Autodesk Inventor part; units mm, degrees
note: some values were not read from the file. Chosen so that the rebuilt part matches the saved one: sketch regions of "LensplateMount".
(part 2 of 2)
sketch "ShorterHoneycomb" plane through (93.9578, 0, 52.0444) normal (1, 0, 0) x (0, 0, -1)
  line L0 (0, 131) -> (119, 131)
  line L1 (119, 131) -> (119, 0)
  line L2 (119, 0) -> (0, 0)
  line L3 (0, 0) -> (0, 131)
  line L4 (7, 131) -> (112, 131)
  line L5 (112, 131) -> (112, 0)
  line L6 (112, 0) -> (7, 0)
  line L7 (7, 0) -> (7, 131)
  line L8 (21.8083, 115) -> (14.3028, 115)
  line L9 (14.3028, 115) -> (10.55, 121.5)
  line L10 (10.55, 121.5) -> (14.3028, 128)
  line L11 (14.3028, 128) -> (21.8083, 128)
  line L12 (21.8083, 128) -> (25.5611, 121.5)
  line L13 (25.5611, 121.5) -> (21.8083, 115)
  line L14 (33.644, 107.5) -> (26.1385, 107.5)
  line L15 (26.1385, 107.5) -> (22.3857, 114)
  line L16 (22.3857, 114) -> (26.1385, 120.5)
  line L17 (26.1385, 120.5) -> (33.644, 120.5)
  line L18 (33.644, 120.5) -> (37.3968, 114)
  line L19 (37.3968, 114) -> (33.644, 107.5)
  line L20 (0, 131) -> (119, 131) projected
  line L21 (25.5611, 121.5) -> (26.1385, 120.5) construction
  line L22 (21.8083, 115) -> (22.3857, 114) construction
  line L23 (21.8083, 100) -> (14.3028, 100)
  line L24 (14.3028, 100) -> (10.55, 106.5)
  line L25 (10.55, 106.5) -> (14.3028, 113)
  line L26 (14.3028, 113) -> (21.8083, 113)
  line L27 (21.8083, 113) -> (25.5611, 106.5)
  line L28 (25.5611, 106.5) -> (21.8083, 100)
  line L29 (33.644, 92.5) -> (26.1385, 92.5)
  line L30 (26.1385, 92.5) -> (22.3857, 99)
  line L31 (22.3857, 99) -> (26.1385, 105.5)
  line L32 (26.1385, 105.5) -> (33.644, 105.5)
  line L33 (33.644, 105.5) -> (37.3968, 99)
  line L34 (37.3968, 99) -> (33.644, 92.5)
  line L35 (25.5611, 106.5) -> (26.1385, 105.5) construction
  line L36 (21.8083, 100) -> (22.3857, 99) construction
  line L37 (21.8083, 85) -> (14.3028, 85)
  line L38 (14.3028, 85) -> (10.55, 91.5)
  line L39 (10.55, 91.5) -> (14.3028, 98)
  line L40 (14.3028, 98) -> (21.8083, 98)
  line L41 (21.8083, 98) -> (25.5611, 91.5)
  line L42 (25.5611, 91.5) -> (21.8083, 85)
  line L43 (33.644, 77.5) -> (26.1385, 77.5)
  line L44 (26.1385, 77.5) -> (22.3857, 84)
  line L45 (22.3857, 84) -> (26.1385, 90.5)
  line L46 (26.1385, 90.5) -> (33.644, 90.5)
  line L47 (33.644, 90.5) -> (37.3968, 84)
  line L48 (37.3968, 84) -> (33.644, 77.5)
  line L49 (25.5611, 91.5) -> (26.1385, 90.5) construction
  line L50 (21.8083, 85) -> (22.3857, 84) construction
  line L51 (21.8083, 70) -> (14.3028, 70)
  line L52 (14.3028, 70) -> (10.55, 76.5)
  line L53 (10.55, 76.5) -> (14.3028, 83)
  line L54 (14.3028, 83) -> (21.8083, 83)
  line L55 (21.8083, 83) -> (25.5611, 76.5)
  line L56 (25.5611, 76.5) -> (21.8083, 70)
  line L57 (33.644, 62.5) -> (26.1385, 62.5)
  line L58 (26.1385, 62.5) -> (22.3857, 69)
  line L59 (22.3857, 69) -> (26.1385, 75.5)
  line L60 (26.1385, 75.5) -> (33.644, 75.5)
  line L61 (33.644, 75.5) -> (37.3968, 69)
  line L62 (37.3968, 69) -> (33.644, 62.5)
  line L63 (25.5611, 76.5) -> (26.1385, 75.5) construction
  line L64 (21.8083, 70) -> (22.3857, 69) construction
  line L65 (21.8083, 55) -> (14.3028, 55)
  line L66 (14.3028, 55) -> (10.55, 61.5)
  line L67 (10.55, 61.5) -> (14.3028, 68)
  line L68 (14.3028, 68) -> (21.8083, 68)
  line L69 (21.8083, 68) -> (25.5611, 61.5)
  line L70 (25.5611, 61.5) -> (21.8083, 55)
  line L71 (33.644, 47.5) -> (26.1385, 47.5)
  line L72 (26.1385, 47.5) -> (22.3857, 54)
  line L73 (22.3857, 54) -> (26.1385, 60.5)
  line L74 (26.1385, 60.5) -> (33.644, 60.5)
  line L75 (33.644, 60.5) -> (37.3968, 54)
  line L76 (37.3968, 54) -> (33.644, 47.5)
  line L77 (25.5611, 61.5) -> (26.1385, 60.5) construction
  line L78 (21.8083, 55) -> (22.3857, 54) construction
  line L79 (21.8083, 40) -> (14.3028, 40)
  line L80 (14.3028, 40) -> (10.55, 46.5)
  line L81 (10.55, 46.5) -> (14.3028, 53)
  line L82 (14.3028, 53) -> (21.8083, 53)
  line L83 (21.8083, 53) -> (25.5611, 46.5)
  line L84 (25.5611, 46.5) -> (21.8083, 40)
  line L85 (33.644, 32.5) -> (26.1385, 32.5)
  line L86 (26.1385, 32.5) -> (22.3857, 39)
  line L87 (22.3857, 39) -> (26.1385, 45.5)
  line L88 (26.1385, 45.5) -> (33.644, 45.5)
  line L89 (33.644, 45.5) -> (37.3968, 39)
  line L90 (37.3968, 39) -> (33.644, 32.5)
  line L91 (25.5611, 46.5) -> (26.1385, 45.5) construction
  line L92 (21.8083, 40) -> (22.3857, 39) construction
  line L93 (21.8083, 25) -> (14.3028, 25)
  line L94 (14.3028, 25) -> (10.55, 31.5)
  line L95 (10.55, 31.5) -> (14.3028, 38)
  line L96 (14.3028, 38) -> (21.8083, 38)
  line L97 (21.8083, 38) -> (25.5611, 31.5)
  line L98 (25.5611, 31.5) -> (21.8083, 25)
  line L99 (33.644, 17.5) -> (26.1385, 17.5)
  line L100 (26.1385, 17.5) -> (22.3857, 24)
  line L101 (22.3857, 24) -> (26.1385, 30.5)
  line L102 (26.1385, 30.5) -> (33.644, 30.5)
  line L103 (33.644, 30.5) -> (37.3968, 24)
  line L104 (37.3968, 24) -> (33.644, 17.5)
  line L105 (25.5611, 31.5) -> (26.1385, 30.5) construction
  line L106 (21.8083, 25) -> (22.3857, 24) construction
  line L107 (21.8083, 10) -> (14.3028, 10)
  line L108 (14.3028, 10) -> (10.55, 16.5)
  line L109 (10.55, 16.5) -> (14.3028, 23)
  line L110 (14.3028, 23) -> (21.8083, 23)
  line L111 (21.8083, 23) -> (25.5611, 16.5)
  line L112 (25.5611, 16.5) -> (21.8083, 10)
  line L113 (33.644, 2.5) -> (26.1385, 2.5)
  line L114 (26.1385, 2.5) -> (22.3857, 9)
  line L115 (22.3857, 9) -> (26.1385, 15.5)
  line L116 (26.1385, 15.5) -> (33.644, 15.5)
  line L117 (33.644, 15.5) -> (37.3968, 9)
  line L118 (37.3968, 9) -> (33.644, 2.5)
  line L119 (25.5611, 16.5) -> (26.1385, 15.5) construction
  line L120 (21.8083, 10) -> (22.3857, 9) construction
  line L121 (45.4833, 115) -> (37.9778, 115)
  line L122 (37.9778, 115) -> (34.225, 121.5)
  line L123 (34.225, 121.5) -> (37.9778, 128)
  line L124 (37.9778, 128) -> (45.4833, 128)
  line L125 (45.4833, 128) -> (49.2361, 121.5)
  line L126 (49.2361, 121.5) -> (45.4833, 115)
  line L127 (57.319, 107.5) -> (49.8135, 107.5)
  line L128 (49.8135, 107.5) -> (46.0607, 114)
  line L129 (46.0607, 114) -> (49.8135, 120.5)
  line L130 (49.8135, 120.5) -> (57.319, 120.5)
  line L131 (57.319, 120.5) -> (61.0718, 114)
  line L132 (61.0718, 114) -> (57.319, 107.5)
  line L133 (49.2361, 121.5) -> (49.8135, 120.5) construction
  line L134 (45.4833, 115) -> (46.0607, 114) construction
  line L135 (45.4833, 100) -> (37.9778, 100)
  line L136 (37.9778, 100) -> (34.225, 106.5)
  line L137 (34.225, 106.5) -> (37.9778, 113)
  line L138 (37.9778, 113) -> (45.4833, 113)
  line L139 (45.4833, 113) -> (49.2361, 106.5)
  line L140 (49.2361, 106.5) -> (45.4833, 100)
  line L141 (57.319, 92.5) -> (49.8135, 92.5)
  line L142 (49.8135, 92.5) -> (46.0607, 99)
  line L143 (46.0607, 99) -> (49.8135, 105.5)
  line L144 (49.8135, 105.5) -> (57.319, 105.5)
  line L145 (57.319, 105.5) -> (61.0718, 99)
  line L146 (61.0718, 99) -> (57.319, 92.5)
  line L147 (49.2361, 106.5) -> (49.8135, 105.5) construction
  line L148 (45.4833, 100) -> (46.0607, 99) construction
  line L149 (45.4833, 85) -> (37.9778, 85)
  line L150 (37.9778, 85) -> (34.225, 91.5)
  line L151 (34.225, 91.5) -> (37.9778, 98)
  line L152 (37.9778, 98) -> (45.4833, 98)
  line L153 (45.4833, 98) -> (49.2361, 91.5)
  line L154 (49.2361, 91.5) -> (45.4833, 85)
  line L155 (57.319, 77.5) -> (49.8135, 77.5)
  line L156 (49.8135, 77.5) -> (46.0607, 84)
  line L157 (46.0607, 84) -> (49.8135, 90.5)
  line L158 (49.8135, 90.5) -> (57.319, 90.5)
  line L159 (57.319, 90.5) -> (61.0718, 84)
  line L160 (61.0718, 84) -> (57.319, 77.5)
  line L161 (49.2361, 91.5) -> (49.8135, 90.5) construction
  line L162 (45.4833, 85) -> (46.0607, 84) construction
  line L163 (45.4833, 70) -> (37.9778, 70)
  line L164 (37.9778, 70) -> (34.225, 76.5)
  line L165 (34.225, 76.5) -> (37.9778, 83)
  line L166 (37.9778, 83) -> (45.4833, 83)
  line L167 (45.4833, 83) -> (49.2361, 76.5)
  line L168 (49.2361, 76.5) -> (45.4833, 70)
  line L169 (57.319, 62.5) -> (49.8135, 62.5)
  line L170 (49.8135, 62.5) -> (46.0607, 69)
  line L171 (46.0607, 69) -> (49.8135, 75.5)
  line L172 (49.8135, 75.5) -> (57.319, 75.5)
  line L173 (57.319, 75.5) -> (61.0718, 69)
  line L174 (61.0718, 69) -> (57.319, 62.5)
  line L175 (49.2361, 76.5) -> (49.8135, 75.5) construction
  line L176 (45.4833, 70) -> (46.0607, 69) construction
  line L177 (45.4833, 55) -> (37.9778, 55)
  line L178 (37.9778, 55) -> (34.225, 61.5)
  line L179 (34.225, 61.5) -> (37.9778, 68)
  line L180 (37.9778, 68) -> (45.4833, 68)
  line L181 (45.4833, 68) -> (49.2361, 61.5)
  line L182 (49.2361, 61.5) -> (45.4833, 55)
  line L183 (57.319, 47.5) -> (49.8135, 47.5)
  line L184 (49.8135, 47.5) -> (46.0607, 54)
  line L185 (46.0607, 54) -> (49.8135, 60.5)
  line L186 (49.8135, 60.5) -> (57.319, 60.5)
  line L187 (57.319, 60.5) -> (61.0718, 54)
  line L188 (61.0718, 54) -> (57.319, 47.5)
  line L189 (49.2361, 61.5) -> (49.8135, 60.5) construction
  line L190 (45.4833, 55) -> (46.0607, 54) construction
  line L191 (45.4833, 40) -> (37.9778, 40)
  line L192 (37.9778, 40) -> (34.225, 46.5)
  line L193 (34.225, 46.5) -> (37.9778, 53)
  line L194 (37.9778, 53) -> (45.4833, 53)
  line L195 (45.4833, 53) -> (49.2361, 46.5)
  line L196 (49.2361, 46.5) -> (45.4833, 40)
  line L197 (57.319, 32.5) -> (49.8135, 32.5)
  line L198 (49.8135, 32.5) -> (46.0607, 39)
  line L199 (46.0607, 39) -> (49.8135, 45.5)
  line L200 (49.8135, 45.5) -> (57.319, 45.5)
  line L201 (57.319, 45.5) -> (61.0718, 39)
  line L202 (61.0718, 39) -> (57.319, 32.5)
  line L203 (49.2361, 46.5) -> (49.8135, 45.5) construction
  line L204 (45.4833, 40) -> (46.0607, 39) construction
  line L205 (45.4833, 25) -> (37.9778, 25)
  line L206 (37.9778, 25) -> (34.225, 31.5)
  line L207 (34.225, 31.5) -> (37.9778, 38)
  line L208 (37.9778, 38) -> (45.4833, 38)
  line L209 (45.4833, 38) -> (49.2361, 31.5)
  line L210 (49.2361, 31.5) -> (45.4833, 25)
  line L211 (57.319, 17.5) -> (49.8135, 17.5)
  line L212 (49.8135, 17.5) -> (46.0607, 24)
  line L213 (46.0607, 24) -> (49.8135, 30.5)
  line L214 (49.8135, 30.5) -> (57.319, 30.5)
  line L215 (57.319, 30.5) -> (61.0718, 24)
  line L216 (61.0718, 24) -> (57.319, 17.5)
  line L217 (49.2361, 31.5) -> (49.8135, 30.5) construction
  line L218 (45.4833, 25) -> (46.0607, 24) construction
  line L219 (45.4833, 10) -> (37.9778, 10)
  line L220 (37.9778, 10) -> (34.225, 16.5)
  line L221 (34.225, 16.5) -> (37.9778, 23)
  line L222 (37.9778, 23) -> (45.4833, 23)
  line L223 (45.4833, 23) -> (49.2361, 16.5)
  line L224 (49.2361, 16.5) -> (45.4833, 10)
  line L225 (57.319, 2.5) -> (49.8135, 2.5)
  line L226 (49.8135, 2.5) -> (46.0607, 9)
  line L227 (46.0607, 9) -> (49.8135, 15.5)
  line L228 (49.8135, 15.5) -> (57.319, 15.5)
  line L229 (57.319, 15.5) -> (61.0718, 9)
  line L230 (61.0718, 9) -> (57.319, 2.5)
  line L231 (49.2361, 16.5) -> (49.8135, 15.5) construction
  line L232 (45.4833, 10) -> (46.0607, 9) construction
  line L233 (69.1583, 115) -> (61.6528, 115)
  line L234 (61.6528, 115) -> (57.9, 121.5)
  line L235 (57.9, 121.5) -> (61.6528, 128)
  line L236 (61.6528, 128) -> (69.1583, 128)
  line L237 (69.1583, 128) -> (72.9111, 121.5)
  line L238 (72.9111, 121.5) -> (69.1583, 115)
  line L239 (80.994, 107.5) -> (73.4885, 107.5)
  line L240 (73.4885, 107.5) -> (69.7357, 114)
  line L241 (69.7357, 114) -> (73.4885, 120.5)
  line L242 (73.4885, 120.5) -> (80.994, 120.5)
  line L243 (80.994, 120.5) -> (84.7468, 114)
  line L244 (84.7468, 114) -> (80.994, 107.5)
  line L245 (72.9111, 121.5) -> (73.4885, 120.5) construction
  line L246 (69.1583, 115) -> (69.7357, 114) construction
  line L247 (69.1583, 100) -> (61.6528, 100)
  line L248 (61.6528, 100) -> (57.9, 106.5)
  line L249 (57.9, 106.5) -> (61.6528, 113)
  line L250 (61.6528, 113) -> (69.1583, 113)
  line L251 (69.1583, 113) -> (72.9111, 106.5)
  line L252 (72.9111, 106.5) -> (69.1583, 100)
  line L253 (80.994, 92.5) -> (73.4885, 92.5)
  line L254 (73.4885, 92.5) -> (69.7357, 99)
  line L255 (69.7357, 99) -> (73.4885, 105.5)
  line L256 (73.4885, 105.5) -> (80.994, 105.5)
  line L257 (80.994, 105.5) -> (84.7468, 99)
  line L258 (84.7468, 99) -> (80.994, 92.5)
  line L259 (72.9111, 106.5) -> (73.4885, 105.5) construction
  line L260 (69.1583, 100) -> (69.7357, 99) construction
  line L261 (69.1583, 85) -> (61.6528, 85)
  line L262 (61.6528, 85) -> (57.9, 91.5)
  line L263 (57.9, 91.5) -> (61.6528, 98)
  line L264 (61.6528, 98) -> (69.1583, 98)
  line L265 (69.1583, 98) -> (72.9111, 91.5)
  line L266 (72.9111, 91.5) -> (69.1583, 85)
  line L267 (80.994, 77.5) -> (73.4885, 77.5)
  line L268 (73.4885, 77.5) -> (69.7357, 84)
  line L269 (69.7357, 84) -> (73.4885, 90.5)
  line L270 (73.4885, 90.5) -> (80.994, 90.5)
  line L271 (80.994, 90.5) -> (84.7468, 84)
  line L272 (84.7468, 84) -> (80.994, 77.5)
  line L273 (72.9111, 91.5) -> (73.4885, 90.5) construction
  line L274 (69.1583, 85) -> (69.7357, 84) construction
  line L275 (69.1583, 70) -> (61.6528, 70)
  line L276 (61.6528, 70) -> (57.9, 76.5)
  line L277 (57.9, 76.5) -> (61.6528, 83)
  line L278 (61.6528, 83) -> (69.1583, 83)
  line L279 (69.1583, 83) -> (72.9111, 76.5)
  line L280 (72.9111, 76.5) -> (69.1583, 70)
  line L281 (80.994, 62.5) -> (73.4885, 62.5)
  line L282 (73.4885, 62.5) -> (69.7357, 69)
  line L283 (69.7357, 69) -> (73.4885, 75.5)
  line L284 (73.4885, 75.5) -> (80.994, 75.5)
  line L285 (80.994, 75.5) -> (84.7468, 69)
  line L286 (84.7468, 69) -> (80.994, 62.5)
  line L287 (72.9111, 76.5) -> (73.4885, 75.5) construction
  line L288 (69.1583, 70) -> (69.7357, 69) construction
  line L289 (69.1583, 55) -> (61.6528, 55)
  line L290 (61.6528, 55) -> (57.9, 61.5)
  line L291 (57.9, 61.5) -> (61.6528, 68)
  line L292 (61.6528, 68) -> (69.1583, 68)
  line L293 (69.1583, 68) -> (72.9111, 61.5)
  line L294 (72.9111, 61.5) -> (69.1583, 55)
  line L295 (80.994, 47.5) -> (73.4885, 47.5)
  line L296 (73.4885, 47.5) -> (69.7357, 54)
  line L297 (69.7357, 54) -> (73.4885, 60.5)
  line L298 (73.4885, 60.5) -> (80.994, 60.5)
  line L299 (80.994, 60.5) -> (84.7468, 54)
  line L300 (84.7468, 54) -> (80.994, 47.5)
  line L301 (72.9111, 61.5) -> (73.4885, 60.5) construction
  line L302 (69.1583, 55) -> (69.7357, 54) construction
  line L303 (69.1583, 40) -> (61.6528, 40)
  line L304 (61.6528, 40) -> (57.9, 46.5)
  line L305 (57.9, 46.5) -> (61.6528, 53)
  line L306 (61.6528, 53) -> (69.1583, 53)
  line L307 (69.1583, 53) -> (72.9111, 46.5)
  line L308 (72.9111, 46.5) -> (69.1583, 40)
  line L309 (80.994, 32.5) -> (73.4885, 32.5)
  line L310 (73.4885, 32.5) -> (69.7357, 39)
  line L311 (69.7357, 39) -> (73.4885, 45.5)
  line L312 (73.4885, 45.5) -> (80.994, 45.5)
  line L313 (80.994, 45.5) -> (84.7468, 39)
  line L314 (84.7468, 39) -> (80.994, 32.5)
  line L315 (72.9111, 46.5) -> (73.4885, 45.5) construction
  line L316 (69.1583, 40) -> (69.7357, 39) construction
  line L317 (69.1583, 25) -> (61.6528, 25)
  line L318 (61.6528, 25) -> (57.9, 31.5)
  line L319 (57.9, 31.5) -> (61.6528, 38)
  line L320 (61.6528, 38) -> (69.1583, 38)
  line L321 (69.1583, 38) -> (72.9111, 31.5)
  line L322 (72.9111, 31.5) -> (69.1583, 25)
  line L323 (80.994, 17.5) -> (73.4885, 17.5)
  line L324 (73.4885, 17.5) -> (69.7357, 24)
  line L325 (69.7357, 24) -> (73.4885, 30.5)
  line L326 (73.4885, 30.5) -> (80.994, 30.5)
  line L327 (80.994, 30.5) -> (84.7468, 24)
  line L328 (84.7468, 24) -> (80.994, 17.5)
  line L329 (72.9111, 31.5) -> (73.4885, 30.5) construction
  line L330 (69.1583, 25) -> (69.7357, 24) construction
  line L331 (69.1583, 10) -> (61.6528, 10)
  line L332 (61.6528, 10) -> (57.9, 16.5)
  line L333 (57.9, 16.5) -> (61.6528, 23)
  line L334 (61.6528, 23) -> (69.1583, 23)
  line L335 (69.1583, 23) -> (72.9111, 16.5)
  line L336 (72.9111, 16.5) -> (69.1583, 10)
  line L337 (80.994, 2.5) -> (73.4885, 2.5)
  line L338 (73.4885, 2.5) -> (69.7357, 9)
  line L339 (69.7357, 9) -> (73.4885, 15.5)
  line L340 (73.4885, 15.5) -> (80.994, 15.5)
  line L341 (80.994, 15.5) -> (84.7468, 9)
  line L342 (84.7468, 9) -> (80.994, 2.5)
  line L343 (72.9111, 16.5) -> (73.4885, 15.5) construction
  line L344 (69.1583, 10) -> (69.7357, 9) construction
  line L345 (92.8333, 115) -> (85.3278, 115)
  line L346 (85.3278, 115) -> (81.575, 121.5)
  line L347 (81.575, 121.5) -> (85.3278, 128)
  line L348 (85.3278, 128) -> (92.8333, 128)
  line L349 (92.8333, 128) -> (96.5861, 121.5)
  line L350 (96.5861, 121.5) -> (92.8333, 115)
  line L351 (104.669, 107.5) -> (97.1635, 107.5)
  line L352 (97.1635, 107.5) -> (93.4107, 114)
  line L353 (93.4107, 114) -> (97.1635, 120.5)
  line L354 (97.1635, 120.5) -> (104.669, 120.5)
  line L355 (104.669, 120.5) -> (108.4218, 114)
  line L356 (108.4218, 114) -> (104.669, 107.5)
  line L357 (96.5861, 121.5) -> (97.1635, 120.5) construction
  line L358 (92.8333, 115) -> (93.4107, 114) construction
  line L359 (92.8333, 100) -> (85.3278, 100)
  line L360 (85.3278, 100) -> (81.575, 106.5)
  line L361 (81.575, 106.5) -> (85.3278, 113)
  line L362 (85.3278, 113) -> (92.8333, 113)
  line L363 (92.8333, 113) -> (96.5861, 106.5)
  line L364 (96.5861, 106.5) -> (92.8333, 100)
  line L365 (104.669, 92.5) -> (97.1635, 92.5)
  line L366 (97.1635, 92.5) -> (93.4107, 99)
  line L367 (93.4107, 99) -> (97.1635, 105.5)
  line L368 (97.1635, 105.5) -> (104.669, 105.5)
  line L369 (104.669, 105.5) -> (108.4218, 99)
  line L370 (108.4218, 99) -> (104.669, 92.5)
  line L371 (96.5861, 106.5) -> (97.1635, 105.5) construction
  line L372 (92.8333, 100) -> (93.4107, 99) construction
  line L373 (92.8333, 85) -> (85.3278, 85)
  line L374 (85.3278, 85) -> (81.575, 91.5)
  line L375 (81.575, 91.5) -> (85.3278, 98)
  line L376 (85.3278, 98) -> (92.8333, 98)
  line L377 (92.8333, 98) -> (96.5861, 91.5)
  line L378 (96.5861, 91.5) -> (92.8333, 85)
  line L379 (104.669, 77.5) -> (97.1635, 77.5)
  line L380 (97.1635, 77.5) -> (93.4107, 84)
  line L381 (93.4107, 84) -> (97.1635, 90.5)
  line L382 (97.1635, 90.5) -> (104.669, 90.5)
  line L383 (104.669, 90.5) -> (108.4218, 84)
  line L384 (108.4218, 84) -> (104.669, 77.5)
  line L385 (96.5861, 91.5) -> (97.1635, 90.5) construction
  line L386 (92.8333, 85) -> (93.4107, 84) construction
  line L387 (92.8333, 70) -> (85.3278, 70)
  line L388 (85.3278, 70) -> (81.575, 76.5)
  line L389 (81.575, 76.5) -> (85.3278, 83)
  line L390 (85.3278, 83) -> (92.8333, 83)
  line L391 (92.8333, 83) -> (96.5861, 76.5)
  line L392 (96.5861, 76.5) -> (92.8333, 70)
  line L393 (104.669, 62.5) -> (97.1635, 62.5)
  line L394 (97.1635, 62.5) -> (93.4107, 69)
  line L395 (93.4107, 69) -> (97.1635, 75.5)
  line L396 (97.1635, 75.5) -> (104.669, 75.5)
  line L397 (104.669, 75.5) -> (108.4218, 69)
  line L398 (108.4218, 69) -> (104.669, 62.5)
  line L399 (96.5861, 76.5) -> (97.1635, 75.5) construction
  line L400 (92.8333, 70) -> (93.4107, 69) construction
  line L401 (92.8333, 55) -> (85.3278, 55)
  line L402 (85.3278, 55) -> (81.575, 61.5)
  line L403 (81.575, 61.5) -> (85.3278, 68)
  line L404 (85.3278, 68) -> (92.8333, 68)
  line L405 (92.8333, 68) -> (96.5861, 61.5)
  line L406 (96.5861, 61.5) -> (92.8333, 55)
  line L407 (104.669, 47.5) -> (97.1635, 47.5)
  line L408 (97.1635, 47.5) -> (93.4107, 54)
  line L409 (93.4107, 54) -> (97.1635, 60.5)
  line L410 (97.1635, 60.5) -> (104.669, 60.5)
  line L411 (104.669, 60.5) -> (108.4218, 54)
  line L412 (108.4218, 54) -> (104.669, 47.5)
  line L413 (96.5861, 61.5) -> (97.1635, 60.5) construction
  line L414 (92.8333, 55) -> (93.4107, 54) construction
  line L415 (92.8333, 40) -> (85.3278, 40)
  line L416 (85.3278, 40) -> (81.575, 46.5)
  line L417 (81.575, 46.5) -> (85.3278, 53)
  line L418 (85.3278, 53) -> (92.8333, 53)
  line L419 (92.8333, 53) -> (96.5861, 46.5)
  line L420 (96.5861, 46.5) -> (92.8333, 40)
  line L421 (104.669, 32.5) -> (97.1635, 32.5)
  line L422 (97.1635, 32.5) -> (93.4107, 39)
  line L423 (93.4107, 39) -> (97.1635, 45.5)
  line L424 (97.1635, 45.5) -> (104.669, 45.5)
  line L425 (104.669, 45.5) -> (108.4218, 39)
  line L426 (108.4218, 39) -> (104.669, 32.5)
  line L427 (96.5861, 46.5) -> (97.1635, 45.5) construction
  line L428 (92.8333, 40) -> (93.4107, 39) construction
  line L429 (92.8333, 25) -> (85.3278, 25)
  line L430 (85.3278, 25) -> (81.575, 31.5)
  line L431 (81.575, 31.5) -> (85.3278, 38)
  line L432 (85.3278, 38) -> (92.8333, 38)
  line L433 (92.8333, 38) -> (96.5861, 31.5)
  line L434 (96.5861, 31.5) -> (92.8333, 25)
  line L435 (104.669, 17.5) -> (97.1635, 17.5)
  line L436 (97.1635, 17.5) -> (93.4107, 24)
  line L437 (93.4107, 24) -> (97.1635, 30.5)
  line L438 (97.1635, 30.5) -> (104.669, 30.5)
  line L439 (104.669, 30.5) -> (108.4218, 24)
  line L440 (108.4218, 24) -> (104.669, 17.5)
  line L441 (96.5861, 31.5) -> (97.1635, 30.5) construction
  line L442 (92.8333, 25) -> (93.4107, 24) construction
  line L443 (92.8333, 10) -> (85.3278, 10)
  line L444 (85.3278, 10) -> (81.575, 16.5)
  line L445 (81.575, 16.5) -> (85.3278, 23)
  line L446 (85.3278, 23) -> (92.8333, 23)
  line L447 (92.8333, 23) -> (96.5861, 16.5)
  line L448 (96.5861, 16.5) -> (92.8333, 10)
  line L449 (104.669, 2.5) -> (97.1635, 2.5)
  line L450 (97.1635, 2.5) -> (93.4107, 9)
  line L451 (93.4107, 9) -> (97.1635, 15.5)
  line L452 (97.1635, 15.5) -> (104.669, 15.5)
  line L453 (104.669, 15.5) -> (108.4218, 9)
  line L454 (108.4218, 9) -> (104.669, 2.5)
  line L455 (96.5861, 16.5) -> (97.1635, 15.5) construction
  line L456 (92.8333, 10) -> (93.4107, 9) construction
  line L457 (116.5083, 115) -> (109.0028, 115)
  line L458 (109.0028, 115) -> (105.25, 121.5)
  line L459 (109.0028, 128) -> (116.5083, 128)
  line L460 (116.5083, 128) -> (120.2611, 121.5)
  line L461 (120.2611, 121.5) -> (116.5083, 115)
  line L462 (105.25, 121.5) -> (109.0028, 128)
  line L463 (116.5083, 100) -> (109.0028, 100)
  line L464 (109.0028, 100) -> (105.25, 106.5)
  line L465 (109.0028, 113) -> (116.5083, 113)
  line L466 (116.5083, 113) -> (120.2611, 106.5)
  line L467 (120.2611, 106.5) -> (116.5083, 100)
  line L468 (105.25, 106.5) -> (109.0028, 113)
  line L469 (116.5083, 85) -> (109.0028, 85)
  line L470 (109.0028, 85) -> (105.25, 91.5)
  line L471 (109.0028, 98) -> (116.5083, 98)
  line L472 (116.5083, 98) -> (120.2611, 91.5)
  line L473 (120.2611, 91.5) -> (116.5083, 85)
  line L474 (105.25, 91.5) -> (109.0028, 98)
  line L475 (116.5083, 70) -> (109.0028, 70)
  line L476 (109.0028, 70) -> (105.25, 76.5)
  line L477 (109.0028, 83) -> (116.5083, 83)
  line L478 (116.5083, 83) -> (120.2611, 76.5)
  line L479 (120.2611, 76.5) -> (116.5083, 70)
  line L480 (105.25, 76.5) -> (109.0028, 83)
  line L481 (116.5083, 55) -> (109.0028, 55)
  line L482 (109.0028, 55) -> (105.25, 61.5)
  line L483 (109.0028, 68) -> (116.5083, 68)
  line L484 (116.5083, 68) -> (120.2611, 61.5)
  line L485 (120.2611, 61.5) -> (116.5083, 55)
  line L486 (105.25, 61.5) -> (109.0028, 68)
  line L487 (116.5083, 40) -> (109.0028, 40)
  line L488 (109.0028, 40) -> (105.25, 46.5)
  line L489 (109.0028, 53) -> (116.5083, 53)
  line L490 (116.5083, 53) -> (120.2611, 46.5)
  line L491 (120.2611, 46.5) -> (116.5083, 40)
  line L492 (105.25, 46.5) -> (109.0028, 53)
  line L493 (116.5083, 25) -> (109.0028, 25)
  line L494 (109.0028, 25) -> (105.25, 31.5)
  line L495 (109.0028, 38) -> (116.5083, 38)
  line L496 (116.5083, 38) -> (120.2611, 31.5)
  line L497 (120.2611, 31.5) -> (116.5083, 25)
  line L498 (105.25, 31.5) -> (109.0028, 38)
  line L499 (116.5083, 10) -> (109.0028, 10)
  line L500 (109.0028, 10) -> (105.25, 16.5)
  line L501 (109.0028, 23) -> (116.5083, 23)
  line L502 (116.5083, 23) -> (120.2611, 16.5)
  line L503 (120.2611, 16.5) -> (116.5083, 10)
  line L504 (105.25, 16.5) -> (109.0028, 23)
  point P0 (52.0444, 0)
  point P1 (18.0556, 121.5)
  point P2 (29.8912, 114)
  point P3 (18.0556, 106.5)
  point P4 (29.8912, 99)
  point P5 (18.0556, 91.5)
  point P6 (29.8912, 84)
  point P7 (18.0556, 76.5)
  point P8 (29.8912, 69)
  point P9 (18.0556, 61.5)
  point P10 (29.8912, 54)
  point P11 (18.0556, 46.5)
  point P12 (29.8912, 39)
  point P13 (18.0556, 31.5)
  point P14 (29.8912, 24)
  point P15 (18.0556, 16.5)
  point P16 (29.8912, 9)
  point P17 (41.7306, 121.5)
  point P18 (53.5662, 114)
  point P19 (41.7306, 106.5)
  point P20 (53.5662, 99)
  point P21 (41.7306, 91.5)
  point P22 (53.5662, 84)
  point P23 (41.7306, 76.5)
  point P24 (53.5662, 69)
  point P25 (41.7306, 61.5)
  point P26 (53.5662, 54)
  point P27 (41.7306, 46.5)
  point P28 (53.5662, 39)
  point P29 (41.7306, 31.5)
  point P30 (53.5662, 24)
  point P31 (41.7306, 16.5)
  point P32 (53.5662, 9)
  point P33 (65.4056, 121.5)
  point P34 (77.2412, 114)
  point P35 (65.4056, 106.5)
  point P36 (77.2412, 99)
  point P37 (65.4056, 91.5)
  point P38 (77.2412, 84)
  point P39 (65.4056, 76.5)
  point P40 (77.2412, 69)
  point P41 (65.4056, 61.5)
  point P42 (77.2412, 54)
  point P43 (65.4056, 46.5)
  point P44 (77.2412, 39)
  point P45 (65.4056, 31.5)
  point P46 (77.2412, 24)
  point P47 (65.4056, 16.5)
  point P48 (77.2412, 9)
  point P49 (89.0806, 121.5)
  point P50 (100.9162, 114)
  point P51 (89.0806, 106.5)
  point P52 (100.9162, 99)
  point P53 (89.0806, 91.5)
  point P54 (100.9162, 84)
  point P55 (89.0806, 76.5)
  point P56 (100.9162, 69)
  point P57 (89.0806, 61.5)
  point P58 (100.9162, 54)
  point P59 (89.0806, 46.5)
  point P60 (100.9162, 39)
  point P61 (89.0806, 31.5)
  point P62 (100.9162, 24)
  point P63 (89.0806, 16.5)
  point P64 (100.9162, 9)
  point P65 (112.7556, 121.5)
  dimension "d32" = 13
  dimension "d33" = 1
  dimension "d35" = 3
  dimension "d36" = 3.55
  dimension "d39" = 15
  dimension "d42" = 23.675
  dimension "d56" = 1
  dimension "d57" = 2
  dimension "d58" = 1
  dimension "d59" = 1.0031
  dimension "d62" = 23.675
  dimension "d137" = 1
  dimension "d138" = 1.0031
  dimension "d139" = 1.0031
  dimension "d140" = 2
  dimension "d141" = 3.5782
  constraints: 1008 end point, 7 parallel, 4 horizontal, 2 collinear, 2 perpendicular, 1 vertical, 991 other
  measures "d32" distance between parallel lines of L8 L11
  measures "d33" distance between parallel lines of L16 L13
  measures "d35" distance between parallel lines of L4 L11
  measures "d36" distance from line of L7 L9.end
  measures "d39" distance of L14.end L29.end
  measures "d42" distance of L14.end L127.end
  measures "d56" distance between parallel lines of L381 L378
  measures "d57" distance between parallel lines of L376 L359
  measures "d58" distance between parallel lines of L366 L377
  measures "d59" distance between parallel lines of L258 L375
  measures "d62" distance of point (89.081, 121.5) point (112.756, 121.5)
  measures "d137" distance between parallel lines of L27 L15
  measures "d138" distance between parallel lines of L137 L19
  measures "d139" distance between parallel lines of L18 L122
  measures "d140" distance between parallel lines of L26 L8
  measures "d141" distance from line of L5 L356.start
extrude "HoneycombShortSide" [suppressed]
extrude "SidePanels" [suppressed]
sketch "DroneAttachmentSide1" plane through (-95.0422, 0, 52.0444) normal (0, 0, 1) x (1, 0, 0)
  circle A0 centre (54.5, 138) radius 3.5
  circle A1 centre (134.5, 138) radius 3.5
  line L0 (54.5, 138) -> (134.5, 138) construction
  line L1 (0, 131) -> (189, 131) projected
  line L2 (54.5, 138) -> (54.5, 131) construction
  line L3 (182, 131) -> (7, 131) projected
  line L4 (134.5, 138) -> (134.5, 131) construction
  line L5 (0, 131) -> (54.5, 138)
  line L6 (134.5, 138) -> (189, 131)
  arc A2 (64.5, 138) -> (44.5815, 136.7261) centre (54.5, 138) ccw
  line L7 (64.5, 138) -> (70.3737, 131)
  line L8 (64.5, 138) -> (73.6379, 138) construction
  line L9 (0, 131) -> (70.3737, 131)
  arc A3 (144.4185, 136.7261) -> (124.5, 138) centre (134.5, 138) ccw
  line L10 (124.5, 138) -> (116.1577, 131)
  line L11 (124.5, 138) -> (130.7015, 138) construction
  line L12 (116.1577, 131) -> (189, 131)
  line L13 (189, 131) -> (0, 131) projected
  line L14 (0, 0) -> (189, 0) projected
  point P0 (95.0422, 0)
  dimension "d72" = 7
  dimension "d73" = 80
  dimension "d74" = 7
  dimension "d75" = 10
  dimension "d76" = 50
  dimension "d77" = 140
  dimension "d133" = 138
  constraints: 22 end point, 6 point on line, 4 centre point, 4 collinear, 4 point on circle, 2 coincident, 2 equal length, 2 equal radius, 2 horizontal, 2 perpendicular, 1 parallel
  measures "d72" diameter of A0
  measures "d73" distance of L0.start L0.end
  measures "d74" distance of L2.end L0.start
  measures "d75" radius of A2
  measures "d76" angle of L7 L8
  measures "d77" angle of L10 L11
  measures "d133" distance from line of L14 A2.centre
extrude "DroneAttachment1" add sketch "DroneAttachmentSide1" against normal blind 4
sketch "Sketch5" plane through (93.9578, 0, -66.9556) normal (0, 0, -1) x (-1, 0, 0)
  circle A0 centre (54.5, 138) radius 3.5 projected
  circle A1 centre (54.5, 138) radius 3.5
  circle A2 centre (134.5, 138) radius 3.5 projected
  circle A3 centre (134.5, 138) radius 3.5
  line L0 (72.8423, 131) -> (0, 131)
  line L1 (0, 131) -> (44.5815, 136.7261)
  line L2 (0, 131) -> (44.5815, 136.7261) projected
  line L3 (72.8423, 131) -> (64.5, 138)
  line L4 (72.8423, 131) -> (64.5, 138) projected
  arc A4 (64.5, 138) -> (44.5815, 136.7261) centre (54.5, 138) ccw
  line L5 (124.5, 138) -> (118.6263, 131)
  line L6 (124.5, 138) -> (118.6263, 131) projected
  line L7 (118.6263, 131) -> (189, 131)
  line L8 (189, 131) -> (144.4185, 136.7261)
  line L9 (189, 131) -> (144.4185, 136.7261) projected
  arc A5 (144.4185, 136.7261) -> (124.5, 138) centre (134.5, 138) ccw
  point P0 (93.9578, 0)
  constraints: 12 end point, 4 centre point, 4 coincident, 4 collinear, 4 point on circle, 2 horizontal
extrude "Droneattachment2" add sketch "Sketch5" against normal blind 4
sketch "PowerButton" plane through (93.9578, 0, 52.0444) normal (1, 0, 0) x (0, 0, -1)
  line L0 (0, 131) -> (119, 131)
  line L1 (119, 131) -> (119, 0)
  line L2 (119, 0) -> (0, 0)
  line L3 (0, 0) -> (0, 131)
  line L4 (7, 131) -> (112, 131)
  line L5 (112, 131) -> (112, 0)
  line L6 (112, 0) -> (7, 0)
  line L7 (7, 0) -> (7, 131)
  circle A0 centre (27, 61) radius 9.5
  point P0 (52.0444, 0)
  dimension "d82" = 19
  dimension "d83" = 20
  dimension "d84" = 70
  constraints: 16 end point, 4 parallel, 2 horizontal, 2 perpendicular, 1 centre point
  measures "d82" diameter of A0
  measures "d83" distance from line of L7 A0.centre
  measures "d84" distance from line of L0 A0.centre
extrude "PowerButtonSupport" add sketch "PowerButton" against normal blind 7 contours A0
hole "PowerButtonHole" at (93.9578, 61, 25.0444) direction (-1, 0, 0) diameter 15.7 depth 20 tip angle 118
extrude "LensplateMount" add sketch "BasicBox" along normal blind 15 contours L3 L58 L0 | L58 L59 L60 L61 L62 L0 | L3 L39 L38 L0 L62 L61 L60 L59 | L40 L18 L26 L19 L27 L44 L2 L3 | L3 L64 L69 L68 L67 L2 L41 L40 | L36 L37 L1 L55 L54 L53 L52 L0 | L65 L2 L67 L68 L69 L64 | L3 L2 L65 | L45 L7 L6 L44 L27 L19 L26 L18 | L52 L53 L54 L55 L56 L0 | L56 L1 L0 | L2 L47 L46 L51 L50 L1 L35 L34 | L2 L49 L50 L51 L46 L47 | L49 L2 L1
extrude "LensplateaAttachment" add sketch "BasicBox" along normal blind 20 contours L3 L58 L0 | L3 L39 L38 L0 L62 L61 L60 L59 | L40 L18 L26 L19 L27 L44 L2 L3 | L3 L64 L69 L68 L67 L2 L41 L40 | L36 L37 L1 L55 L54 L53 L52 L0 | L3 L2 L65 | L45 L7 L6 L44 L27 L19 L26 L18 | L56 L1 L0 | L2 L47 L46 L51 L50 L1 L35 L34 | L49 L2 L1
sketch "stuffplate_Mount" plane through (-95.0422, 0, 52.0444) normal (0, 0, 1) x (1, 0, 0)
  line L0 (0, 131) -> (189, 131)
  line L1 (189, 0) -> (0, 0)
  line L2 (0, 106) -> (189, 106)
  line L3 (0, 98) -> (189, 98)
  circle A0 centre (81, 102) radius 3
  circle A1 centre (141, 102) radius 3
  line L4 (81, 102) -> (141, 102) construction
  line L5 (141, 102) -> (189, 102) construction
  line L6 (81, 102) -> (0, 102) construction
  line L7 (81, 102) -> (81, 98) construction
  line L8 (81, 102) -> (81, 106) construction
  line L9 (141, 102) -> (141, 106) construction
  line L10 (141, 102) -> (141, 98) construction
  point P0 (95.0422, 0)
  dimension "d111" = 8
  dimension "d112" = 6
  dimension "d116" = 48
  dimension "d117" = 60
  dimension "d118" = 81
  dimension "d119" = 25
  constraints: 22 end point, 6 point on line, 2 centre point, 2 equal length, 2 horizontal, 2 parallel, 1 equal radius, 1 perpendicular
  measures "d111" distance between parallel lines of L3 L2
  measures "d112" diameter of A0
  measures "d116" distance of L2.end L9.end
  measures "d117" distance of L8.end L9.end
  measures "d118" distance of L8.end L2.start
  measures "d119" distance between parallel lines of L0 L2
extrude "StuffplateMount" [suppressed]
sketch "Sketch8" plane through (93.9578, 0, -66.9556) normal (0, 0, -1) x (-1, 0, 0)
  line L0 (179, 106) -> (4, 106)
  line L1 (4, 106) -> (4, 98)
  line L2 (4, 98) -> (179, 98)
  line L3 (179, 98) -> (179, 106)
  point P0 (93.9578, 0)
  dimension "d122" = 8
  dimension "d123" = 175
  constraints: 8 end point, 2 parallel, 1 horizontal, 1 perpendicular
  measures "d122" distance between parallel lines of L2 L0
  measures "d123" distance between parallel lines of L3 L1
extrude "StuffplateMount2" [suppressed]
hole "Hole2" at (-95.0422, 131, 52.0444) at (93.9578, 0, 52.0444) at (-14.0422, 102, 52.0444) at (45.9578, 102, 52.0444) direction (0, 0, -1) diameter 2 end through all
body "Solid1"
